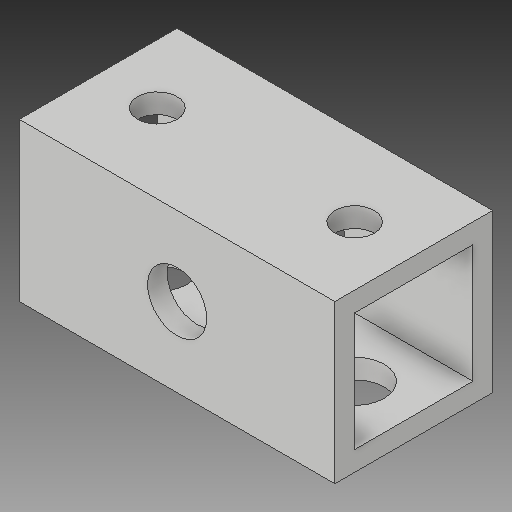
# Autodesk Inventor part: 15102898-16-A-0202
Saved by Autodesk Inventor 2017 (Build 210142000, 142)
## iProperties
Created: 2016-09-26
Part Number: 15102898-16-A-0202
Material: Generic
Document SubType Name: Modeling
Designer: gus
Density: 1 g/cm^3
Appearance: Default
Author: gus
Autodesk Inventor part; units mm, degrees
ref_plane "YZ Plane" through (0, 0, 0) normal (1, 0, 0) x (0, 1, 0)
ref_plane "XZ Plane" through (0, 0, 0) normal (0, 1, 0) x (-1, 0, 0)
ref_plane "XY Plane" through (0, 0, 0) normal (0, 0, 1) x (1, 0, 0)
sketch "Sketch1" plane through (0, 0, 0) normal (1, 0, 0) x (0, 1, 0)
  line L0 (0, 0) -> (-25.4, 0)
  line L1 (-25.4, 0) -> (-25.4, -25.4)
  line L2 (-25.4, -25.4) -> (0, -25.4)
  line L3 (0, -25.4) -> (0, 0)
  line L4 (-3.175, -22.225) -> (-22.225, -22.225)
  line L5 (-22.225, -22.225) -> (-22.225, -3.175)
  line L6 (-22.225, -3.175) -> (-3.175, -3.175)
  line L7 (-3.175, -3.175) -> (-3.175, -22.225)
  dimension "d0" = 25.4
  dimension "d1" = 25.4
  dimension "d2" = 3.175
  constraints: 16 end point, 4 parallel, 2 perpendicular, 1 horizontal, 3 other
  measures "d0" distance of L2.end L1.end
  measures "d1" distance of L1.end L0.end
  measures "d2" distance between parallel lines of L2 L4
extrude "Extrusion1" add sketch "Sketch1" along normal blind 50.8
sketch "Sketch2" plane through (0, -25.4, 0) normal (0, 0, 1) x (1, 0, 0)
  circle A0 centre (25.4, 12.7) radius 4.7625
  line L0 (0, 25.4) -> (50.8, 25.4) projected
  line L1 (0, 25.4) -> (0, 0) projected
  dimension "d5" = 9.525
  dimension "d6" = 12.7
  dimension "d7" = 25.4
  constraints: 1 centre point
  measures "d5" diameter of A0
  measures "d6" distance from line of L0 A0.centre
  measures "d7" distance from line of L1 A0.centre
extrude "Extrusion2" cut sketch "Sketch2" against normal blind 50.8
sketch "Sketch3" plane through (0, 0, 0) normal (0, 1, 0) x (1, 0, 0)
  circle A0 centre (41.275, 12.7) radius 3.175
  circle A1 centre (9.525, 12.7) radius 3.175
  line L0 (50.8, 25.4) -> (50.8, 0) projected
  line L1 (0, 25.4) -> (50.8, 25.4) projected
  line L2 (0, 22.225) -> (0, 3.175) projected
  point P0 (0, 0)
  dimension "d10" = 6.35
  dimension "d11" = 6.35
  dimension "d12" = 9.525
  dimension "d13" = 12.7
  dimension "d14" = 9.525
  dimension "d15" = 12.7
  constraints: 2 centre point
  measures "d10" diameter of A0
  measures "d11" diameter of A1
  measures "d12" distance from line of A0.centre L0
  measures "d13" distance from line of L1 A1.centre
  measures "d14" distance from line of L2 A1.centre
  measures "d15" distance from line of L1 A0.centre
extrude "Extrusion3" cut sketch "Sketch3" against normal blind 3.175
sketch "Sketch4" plane through (0, -25.4, -25.4) normal (0, -1, 0) x (1, 0, 0)
  circle A0 centre (41.275, 12.7) radius 3.175 projected
  circle A1 centre (41.275, 12.7) radius 4.7625
  circle A2 centre (9.525, 12.7) radius 4.7625
  line L0 (0, 25.4) -> (0, 0) projected
  line L1 (0, 0) -> (50.8, 0) projected
  dimension "d18" = 9.525
  dimension "d19" = 9.525
  dimension "d20" = 9.525
  dimension "d21" = 12.7
  constraints: 2 centre point, 1 coincident
  measures "d18" diameter of A1
  measures "d19" diameter of A2
  measures "d20" distance from line of L0 A2.centre
  measures "d21" distance from line of L1 A2.centre
extrude "Extrusion4" cut sketch "Sketch4" against normal blind 3.175 contours A0 | A1 | A2
body "Solid1"
